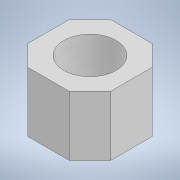
# Autodesk Inventor part: dummy gopro nickle holder
Saved by Autodesk Inventor 2020 (Build 240168000, 168)
## iProperties
Created: 2021-05-10
Part Number: dummy gopro nickle holder
Material: Generic
Document SubType Name: Modeling
Designer: Steven
Density: 1 g/cm^3
Appearance: Default
Author: Steven
Autodesk Inventor part; units mm, degrees
ref_plane "YZ Plane" through (0, 0, 0) normal (1, 0, 0) x (0, 1, 0)
ref_plane "XZ Plane" through (0, 0, 0) normal (0, 1, 0) x (-1, 0, 0)
ref_plane "XY Plane" through (0, 0, 0) normal (0, 0, 1) x (1, 0, 0)
sketch "Sketch1" plane through (0, 0, 0) normal (0, 1, 0) x (-1, 0, 0)
  line L0 (0, 0) -> (0, -16.875) construction
  line L1 (0, -33.75) -> (16.875, -33.75) construction
  line L2 (33.75, -33.75) -> (33.75, -16.875) construction
  line L3 (33.75, 0) -> (16.875, 0) construction
  line L4 (33.75, -16.875) -> (0, -16.875) construction
  line L5 (16.875, -33.75) -> (16.875, 0) construction
  circle A0 centre (16.875, -16.875) radius 10.62
  line L6 (33.75, -16.875) -> (33.75, 0) construction
  line L7 (16.875, 0) -> (0, 0) construction
  line L8 (0, -16.875) -> (0, -33.75) construction
  line L9 (16.875, -33.75) -> (33.75, -33.75) construction
  line L10 (33.75, -25.3125) -> (25.3125, -33.75)
  line L11 (8.4375, -33.75) -> (0, -25.3125)
  line L12 (0, -8.4375) -> (8.4375, 0)
  line L13 (25.3125, 0) -> (33.75, -8.4375)
  line L14 (8.4375, 0) -> (25.3125, 0)
  line L15 (33.75, -8.4375) -> (33.75, -25.3125)
  line L16 (25.3125, -33.75) -> (8.4375, -33.75)
  line L17 (0, -25.3125) -> (0, -8.4375)
  dimension "d0" = 33.75
  dimension "d1" = 33.75
  dimension "d2" = 21.24
  constraints: 36 end point, 9 midpoint, 9 perpendicular, 6 equal length, 2 vertical, 1 centre point, 1 horizontal
  measures "d0" distance of L0.start L1.start
  measures "d1" distance of L1.start L2.start
  measures "d2" diameter of A0
extrude "Extrusion1" add sketch "Sketch1" along normal blind 24.4
sketch "Sketch2" plane through (0, 0, 0) normal (0, -1, 0) x (1, 0, 0)
  circle A0 centre (-16.875, -16.875) radius 10.62 projected
  point P0 (0, 0)
extrude "Extrusion2" add sketch "Sketch2" against normal blind 4
body "Solid1"
